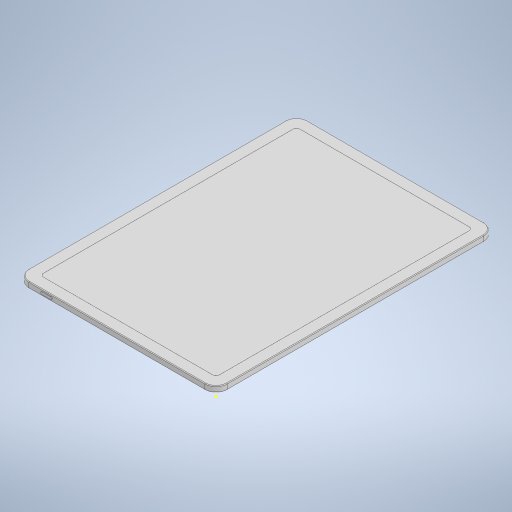
# Autodesk Inventor part: ipad
Saved by Autodesk Inventor 2024.3 (Build 283343000, 343)
## iProperties
Created: 2024-08-06
Part Number: ipad
Material: 일반
Document SubType Name: Modeling
Designer: naru4
Density: 1 g/cm^3
Appearance: 기본값
Author: naru4
Autodesk Inventor part; units mm, degrees
ref_plane "YZ Plane" through (0, 0, 0) normal (1, 0, 0) x (0, 1, 0)
ref_plane "XZ Plane" through (0, 0, 0) normal (0, 1, 0) x (-1, 0, 0)
ref_plane "XY Plane" through (0, 0, 0) normal (0, 0, 1) x (1, 0, 0)
sketch "스케치1" plane through (0, 0, 0) normal (0, 1, 0) x (-1, 0, 0)
  point P0 (0, 0)
sketch "스케치2" plane through (0, 0, 0) normal (0, 1, 0) x (-1, 0, 0)
  line L0 (10, 0) -> (167.5, 0)
  line L1 (177.5, -10) -> (177.5, -239.5)
  line L2 (167.5, -249.5) -> (10, -249.5)
  line L3 (0, -239.5) -> (0, -10)
  arc A0 (177.5, -10) -> (167.5, 0) centre (167.5, -10) ccw
  arc A1 (10, 0) -> (0, -10) centre (10, -10) ccw
  arc A2 (0, -239.5) -> (10, -249.5) centre (10, -239.5) ccw
  arc A3 (167.5, -249.5) -> (177.5, -239.5) centre (167.5, -239.5) ccw
  point P0 (0, 0)
  point P1 (177.5, -249.5)
  point P2 (177.5, 0)
  point P3 (0, -249.5)
  dimension "d19" = 177.5
  dimension "d20" = 249.5
  dimension "d21" = 10
  constraints: 8 end point, 8 point on circle, 8 point on line, 8 tangent, 4 centre point, 3 equal radius, 2 parallel, 1 horizontal, 1 perpendicular
  measures "d19" distance of point (177.5, -249.5) point (0, -249.5)
  measures "d20" distance of point (177.5, 0) point (177.5, -249.5)
  measures "d21" radius of A0
extrude "돌출1" add sketch "스케치2" along normal blind 5.3
fillet "모깎기1" radius 0.6 8 edges at (-2.9289, 5.3, -246.5711) (-88.75, 5.3, -249.5) (-174.5711, 5.3, -246.5711) (-177.5, 5.3, -124.75) (-174.5711, 5.3, -2.9289) (-88.75, 5.3, 0) (-2.9289, 5.3, -2.9289) (0, 5.3, -124.75)
fillet "모깎기2" radius 0.6 8 edges at (-2.9289, 0, -246.5711) (-88.75, 0, -249.5) (-174.5711, 0, -246.5711) (-177.5, 0, -124.75) (-174.5711, 0, -2.9289) (-88.75, 0, 0) (-2.9289, 0, -2.9289) (0, 0, -124.75)
sketch "스케치3" plane through (-167.5, 4.7, 0) normal (0, 0, 1) x (1, 0, 0)
  line L0 (0, -4.1) -> (0, 0) projected
  line L1 (11, -2.05) -> (11, -1.05)
  line L2 (11, -2.05) -> (11, -2.05)
  line L3 (12, -3.05) -> (20, -3.05)
  line L4 (21, -2.05) -> (21, -2.05)
  line L5 (20, -1.05) -> (12, -1.05)
  arc A0 (12, -1.05) -> (11, -2.05) centre (12, -2.05) ccw
  arc A1 (11, -2.05) -> (12, -3.05) centre (12, -2.05) ccw
  arc A2 (20, -3.05) -> (21, -2.05) centre (20, -2.05) ccw
  arc A3 (21, -2.05) -> (20, -1.05) centre (20, -2.05) ccw
  point P0 (167.5, -4.7)
  point P1 (11, -3.05)
  point P2 (21, -3.05)
  point P3 (11, -2.05)
  point P4 (21, -2.05)
  dimension "d29" = 10
  dimension "d30" = 1
  constraints: 10 end point, 8 point on circle, 8 tangent, 7 point on line, 4 centre point, 3 equal radius, 3 perpendicular
  measures "d29" distance of point (11, -3.05) point (21, -3.05)
  measures "d30" radius of A0
extrude "돌출2" add sketch "스케치3" along normal blind 0.5
sketch "스케치4" plane through (0, 5.3, 0) normal (0, 1, 0) x (1, 0, 0)
  line L0 (-176.9, 239.5) -> (-176.9, 10) projected
  line L1 (-0.6, 239.5) -> (-0.6, 10) projected
  line L2 (-164.5, 10) -> (-13, 10)
  arc A0 (-176.9, 10) -> (-167.5, 0.6) centre (-167.5, 10) ccw projected
  arc A1 (-167.5, 248.9) -> (-176.9, 239.5) centre (-167.5, 239.5) ccw projected
  line L3 (-167.5, 13) -> (-167.5, 236.5)
  line L4 (-164.5, 239.5) -> (-13, 239.5)
  line L5 (-167.5, 248.9) -> (-10, 248.9) projected
  line L6 (-10, 236.5) -> (-10, 13)
  arc A2 (-164.5, 239.5) -> (-167.5, 236.5) centre (-164.5, 236.5) ccw
  arc A3 (-10, 236.5) -> (-13, 239.5) centre (-13, 236.5) ccw
  arc A4 (-167.5, 13) -> (-164.5, 10) centre (-164.5, 13) ccw
  arc A5 (-13, 10) -> (-10, 13) centre (-13, 13) ccw
  point P0 (0, 0)
  dimension "d33" = 3
  constraints: 8 end point, 8 point on circle, 8 tangent, 4 centre point, 3 equal radius, 2 horizontal, 2 vertical
  measures "d33" radius of A2
extrude "돌출3" cut sketch "스케치4" against normal blind 0.02
sketch "스케치5" plane through (0, 0, 0) normal (0, -1, 0) x (1, 0, 0)
  arc A0 (-167.5, -0.6) -> (-176.9, -10) centre (-167.5, -10) ccw projected
  line L0 (-165.85, -7.65) -> (-154.6582, -7.65)
  line L1 (-149.85, -12.4582) -> (-149.85, -22.8418)
  line L2 (-154.6582, -27.65) -> (-165.85, -27.65)
  line L3 (-170.6582, -22.8418) -> (-170.6582, -12.4582)
  arc A1 (-154.6582, -27.65) -> (-149.85, -22.8418) centre (-154.6582, -22.8418) ccw
  arc A2 (-149.85, -12.4582) -> (-154.6582, -7.65) centre (-154.6582, -12.4582) ccw
  arc A3 (-165.85, -7.65) -> (-170.6582, -12.4582) centre (-165.85, -12.4582) ccw
  arc A4 (-170.6582, -22.8418) -> (-165.85, -27.65) centre (-165.85, -22.8418) ccw
  circle A5 centre (-165.85, -12.4582) radius 2.75
  circle A6 centre (-165.85, -22.8418) radius 2.75
  line L4 (-154.6582, -22.8418) -> (-154.6582, -12.4582)
  circle A7 centre (-154.6582, -17.65) radius 2.4059
  point P0 (0, 0)
  dimension "d42" = 5.5
  dimension "d43" = 5.5
  constraints: 10 end point, 8 point on circle, 8 tangent, 7 centre point, 3 equal radius, 2 coincident, 2 perpendicular, 2 vertical, 1 horizontal, 1 midpoint
  measures "d42" diameter of A5
  measures "d43" diameter of A6
extrude "돌출4" add sketch "스케치5" along normal blind 0.5
sketch "스케치6" plane through (-154.6582, 0, -17.65) normal (0, -1, 0) x (1, 0, 0)
  circle A0 centre (0, 0) radius 2.4059
  point P0 (154.6582, 17.65)
  constraints: 1 centre point
extrude "돌출5" add sketch "스케치6" along normal blind 0.3
sketch "스케치7" plane through (-165.85, 0, -22.8418) normal (0, -1, 0) x (1, 0, 0)
  circle A0 centre (0, 0) radius 2.75
  point P0 (165.85, 22.8418)
  constraints: 1 centre point
extrude "돌출6" add sketch "스케치7" along normal blind 0.7
sketch "스케치8" plane through (-165.85, 0, -12.4582) normal (0, -1, 0) x (1, 0, 0)
  circle A0 centre (0, 0) radius 2.75
  point P0 (165.85, 12.4582)
  constraints: 1 centre point
extrude "돌출7" add sketch "스케치8" along normal blind 0.7
sketch "스케치9" plane through (-165.85, -0.7, -22.8418) normal (0, -1, 0) x (1, 0, 0)
  circle A0 centre (0, 0) radius 2.25
  point P0 (165.85, 22.8418)
  dimension "d52" = 4.5
  constraints: 1 centre point
  measures "d52" diameter of A0
extrude "돌출8" cut sketch "스케치9" against normal blind 0.1
sketch "스케치10" plane through (-165.85, -0.7, -12.4582) normal (0, -1, 0) x (1, 0, 0)
  circle A0 centre (0, 0) radius 2.25
  point P0 (165.85, 12.4582)
  dimension "d55" = 4.5
  constraints: 1 centre point
  measures "d55" diameter of A0
extrude "돌출9" cut sketch "스케치10" against normal blind 0.1
sketch "스케치11" plane through (-10, 4.7, -249.5) normal (0, 0, -1) x (-1, 0, 0)
  line L0 (0, -4.1) -> (0, 0) projected
  line L1 (157.5, -4.1) -> (157.5, 0) projected
  line L2 (77.75, -3.05) -> (81.75, -3.05)
  line L3 (81.75, -3.05) -> (75.75, -3.05)
  line L4 (74.75, -2.05) -> (74.75, -2.05)
  line L5 (75.75, -1.05) -> (81.75, -1.05)
  line L6 (82.75, -2.05) -> (82.75, -2.05)
  line L7 (0, -2.05) -> (74.75, -2.05)
  line L8 (82.75, -2.05) -> (157.5, -2.05)
  arc A0 (75.75, -1.05) -> (74.75, -2.05) centre (75.75, -2.05) ccw
  arc A1 (74.75, -2.05) -> (75.75, -3.05) centre (75.75, -2.05) ccw
  arc A2 (81.75, -3.05) -> (82.75, -2.05) centre (81.75, -2.05) ccw
  arc A3 (82.75, -2.05) -> (81.75, -1.05) centre (81.75, -2.05) ccw
  point P0 (-10, -4.7)
  point P1 (74.75, -2.05)
  constraints: 14 end point, 8 point on circle, 8 tangent, 4 centre point, 4 midpoint, 4 perpendicular, 3 equal radius
extrude "돌출10" cut sketch "스케치11" against normal blind 8
sketch "스케치12" plane through (-10, 4.7, -241.5) normal (0, 0, -1) x (-1, 0, 0)
  arc A0 (75.75, -1.05) -> (75.75, -3.05) centre (75.75, -2.05) ccw projected
  line L0 (75.75, -1.05) -> (81.75, -1.05) projected
  line L1 (76.75, -2.05) -> (76.75, -1.95)
  line L2 (0, -4.1) -> (157.5, -4.1) projected
  line L3 (76.85, -1.85) -> (80.65, -1.85)
  line L4 (80.75, -1.95) -> (80.75, -2.15)
  line L5 (80.65, -2.25) -> (76.85, -2.25)
  line L6 (76.75, -2.15) -> (76.75, -2.05)
  arc A1 (80.75, -1.95) -> (80.65, -1.85) centre (80.65, -1.95) ccw
  arc A2 (80.65, -2.25) -> (80.75, -2.15) centre (80.65, -2.15) ccw
  arc A3 (76.75, -2.15) -> (76.85, -2.25) centre (76.85, -2.15) ccw
  arc A4 (76.85, -1.85) -> (76.75, -1.95) centre (76.85, -1.95) ccw
  point P0 (-10, -4.7)
  constraints: 10 end point, 8 point on circle, 8 tangent, 4 centre point, 3 equal radius, 3 perpendicular, 1 collinear, 1 parallel
extrude "돌출11" add sketch "스케치12" along normal blind 6
sketch "스케치13" plane through (-10, 4.7, -249.5) normal (0, 0, -1) x (-1, 0, 0)
  line L0 (74.4634, -2.2843) -> (39.4634, -2.2843)
  circle A0 centre (39.4634, -2.2843) radius 0.75
  circle A1 centre (37.4634, -2.2843) radius 0.75
  circle A2 centre (35.4634, -2.2843) radius 0.75
  circle A3 centre (33.4634, -2.2843) radius 0.75
  circle A4 centre (31.4634, -2.2843) radius 0.75
  circle A5 centre (29.4634, -2.2843) radius 0.75
  circle A6 centre (27.4634, -2.2843) radius 0.75
  circle A7 centre (25.4634, -2.2843) radius 0.75
  circle A8 centre (23.4634, -2.2843) radius 0.75
  circle A9 centre (21.4634, -2.2843) radius 0.75
  circle A10 centre (19.4634, -2.2843) radius 0.75
  point P0 (-10, -4.7)
  dimension "d73" = 35
  dimension "d84" = 1.5
  constraints: 11 centre point, 2 end point, 1 coincident, 1 horizontal
  measures "d73" distance of L0.start L0.end
  measures "d84" diameter of A0
extrude "돌출12" cut sketch "스케치13" against normal blind 6
sketch "스케치14" plane through (-10, 4.7, -249.5) normal (0, 0, -1) x (-1, 0, 0)
  arc A0 (81.75, -3.05) -> (81.75, -1.05) centre (81.75, -2.05) ccw projected
  circle A1 centre (117.75, -2.05) radius 0.75
  circle A2 centre (119.75, -2.05) radius 0.75
  circle A3 centre (121.75, -2.05) radius 0.75
  circle A4 centre (123.75, -2.05) radius 0.75
  circle A5 centre (125.75, -2.05) radius 0.75
  circle A6 centre (127.75, -2.05) radius 0.75
  circle A7 centre (129.75, -2.05) radius 0.75
  circle A8 centre (137.75, -2.05) radius 0.75
  circle A9 centre (135.75, -2.05) radius 0.75
  circle A10 centre (133.75, -2.05) radius 0.75
  circle A11 centre (131.75, -2.05) radius 0.77
  point P0 (-10, -4.7)
  constraints: 11 centre point
extrude "돌출13" cut sketch "스케치14" against normal blind 6
fillet "모깎기3" radius 0.3 8 edges at (-169.2499, 0, -9.0583) (-160.2541, 0, -7.65) (-151.2583, 0, -9.0583) (-149.85, 0, -17.65) (-151.2583, 0, -26.2417) (-160.2541, 0, -27.65) (-169.2499, 0, -26.2417) (-170.6582, 0, -17.65)
